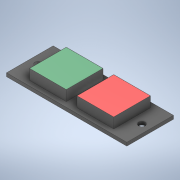
# Autodesk Inventor part: StartStopSwitch
Saved by Autodesk Inventor 2020.4 (Build 244396000, 396)
## iProperties
Created: 2022-03-29
Part Number: StartStopSwitch
Material: 一般
Document SubType Name: Modeling
Designer: Masato Kubotera
Density: 1 g/cm^3
Appearance: 滑らか - 黒
Author: Masato Kubotera
Autodesk Inventor part; units mm, degrees
ref_plane "YZ Plane" through (0, 0, 0) normal (1, 0, 0) x (0, 1, 0)
ref_plane "XZ Plane" through (0, 0, 0) normal (0, 1, 0) x (-1, 0, 0)
ref_plane "XY Plane" through (0, 0, 0) normal (0, 0, 1) x (1, 0, 0)
derived "Cockpit_top_frame.ipt"
sketch "スケッチ3" plane through (0, 0, -22.5) normal (0, 0, 1) x (1, 0, 0)
  line L0 (-86, -140) -> (-52.5, -140) construction
  line L1 (-52.5, -140) -> (-52.5, 5) construction
  line L2 (-52.5, 5) -> (-86, 5) construction
  line L3 (-86, 5) -> (-86, -140) construction
  line L4 (-86, -140) -> (-52.5, 5) construction
  line L5 (-52.5, -140) -> (-86, 5) construction
  line L6 (-73.25, 2.5) -> (-65.25, 2.5) construction
  line L7 (-65.25, 2.5) -> (-65.25, 0) construction
  line L8 (-65.25, 0) -> (-73.25, 0) construction
  line L9 (-73.25, 0) -> (-73.25, 2.5) construction
  line L10 (-73.25, 2.5) -> (-65.25, 0) construction
  line L11 (-65.25, 2.5) -> (-73.25, 0) construction
  line L12 (-81.05, 5) -> (-81.05, 0) construction
  line L13 (-81.05, 0) -> (-86, 0) construction
  arc A0 (-82.5349, 0) -> (-81.05, 1.4849) centre (-81.7925, 0.7425) ccw construction
  line L14 (-73.3, 2.55) -> (-65.2, 2.55) construction
  line L15 (-65.2, 2.55) -> (-65.2, -0.05) construction
  line L16 (-65.2, -0.05) -> (-73.3, -0.05) construction
  line L17 (-73.3, -0.05) -> (-73.3, 2.55) construction
  line L18 (-73.3, 2.55) -> (-65.2, -0.05) construction
  line L19 (-65.2, 2.55) -> (-73.3, -0.05) construction
  line L20 (-73.25, 1.25) -> (-65.25, 1.25) construction
  line L21 (-69.25, 2.5) -> (-69.25, 0) construction
  arc A1 (-71.8151, 2.55) -> (-73.3, 1.0651) centre (-72.5575, 1.8075) ccw construction
  arc A2 (-73.3, -0.05) -> (-71.2, -0.05) centre (-72.25, -0.05) ccw construction
  arc A3 (-65.2, 1.0651) -> (-66.6849, 2.55) centre (-65.9425, 1.8075) ccw construction
  arc A4 (-67.3, -0.05) -> (-65.2, -0.05) centre (-66.25, -0.05) ccw construction
  line L22 (-59.3142, -46.1342) -> (-79.1858, -66.0058) construction
  arc A5 (-61.3142, -66.0058) -> (-59.3142, -64.0058) centre (-61.3142, -64.0058) ccw construction
  line L23 (-69.25, -56.07) -> (-69.25, -78.93) construction
  arc A6 (-77.1858, -46.1342) -> (-79.1858, -48.1342) centre (-77.1858, -48.1342) ccw construction
  arc A7 (-59.3142, -48.1342) -> (-61.3142, -46.1342) centre (-61.3142, -48.1342) ccw construction
  line L24 (-77.1858, -66.0058) -> (-61.3142, -66.0058) construction
  line L25 (-59.9, -65.42) -> (-78.6, -65.42) construction
  line L26 (-59.3142, -64.0058) -> (-59.3142, -48.1342) construction
  line L27 (-79.1858, -48.1342) -> (-79.1858, -64.0058) construction
  line L28 (-78.6, -65.42) -> (-78.6, -46.72) construction
  line L29 (-78.6, -46.72) -> (-59.9, -46.72) construction
  line L30 (-78.6, -65.42) -> (-59.9, -46.72) construction
  line L31 (-59.9, -65.42) -> (-78.6, -46.72) construction
  line L32 (-59.9, -46.72) -> (-59.9, -65.42) construction
  line L33 (-79.1858, -46.1342) -> (-59.3142, -66.0058) construction
  arc A8 (-79.1858, -64.0058) -> (-77.1858, -66.0058) centre (-77.1858, -64.0058) ccw construction
  line L34 (-61.3142, -46.1342) -> (-77.1858, -46.1342) construction
  line L35 (-86, -67.5) -> (-52.5, -67.5) construction
  circle A9 centre (-77.125, 2.5) radius 1.6 construction
  circle A10 centre (-61.375, 2.5) radius 1.6 construction
  line L36 (-80.5, -96.5) -> (-58, -96.5)
  line L37 (-58, -96.5) -> (-58, -38.5)
  line L38 (-58, -38.5) -> (-80.5, -38.5)
  line L39 (-80.5, -38.5) -> (-80.5, -96.5)
  line L40 (-80.5, -96.5) -> (-58, -38.5) construction
  line L41 (-58, -96.5) -> (-80.5, -38.5) construction
  line L42 (-78.1, -47.22) -> (-60.4, -47.22)
  line L43 (-60.4, -47.22) -> (-60.4, -64.92)
  line L44 (-60.4, -64.92) -> (-78.1, -64.92)
  line L45 (-78.1, -64.92) -> (-78.1, -47.22)
  line L46 (-78.1, -47.22) -> (-60.4, -64.92) construction
  line L47 (-60.4, -47.22) -> (-78.1, -64.92) construction
  circle A11 centre (-69.25, -42.5) radius 1.6
  circle A12 centre (-69.25, -42.5) radius 2 construction
  line L48 (-60.4, -70.08) -> (-78.1, -70.08)
  line L49 (-60.4, -87.78) -> (-60.4, -70.08)
  line L50 (-78.1, -87.78) -> (-60.4, -87.78)
  line L51 (-78.1, -70.08) -> (-78.1, -87.78)
  circle A13 centre (-69.25, -92.5) radius 2 construction
  circle A14 centre (-69.25, -92.5) radius 1.6
  circle A15 centre (-69.25, -42.5) radius 3.5 construction
  point P0 (0, 0)
  point P1 (-69.25, -67.5)
  point P2 (-52.5, 0)
  point P3 (-69.25, 1.25)
  point P4 (-81, 0)
  point P5 (-81, 0)
  point P6 (-81, 0)
  point P7 (-69.25, -67.5)
  point P8 (-68.25, -67.5)
  point P9 (-69.25, -67.5)
  point P10 (-77.125, 0)
  point P11 (-77.125, 0)
  point P12 (-61.375, 0)
  point P13 (-61.375, 0)
  point P14 (-61.375, 0)
  point P15 (-69.25, -67.5)
extrude "押し出し1" add sketch "スケッチ3" against normal blind 1.6 contours L39 L38 L37 L36 | L42 L43 L44 L45 | L49 L50 L51 L48
extrude "押し出し2" add sketch "スケッチ3" along normal blind 5 contours L42 L43 L44 L45 | L49 L50 L51 L48
